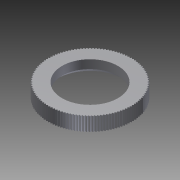
# Autodesk Inventor part: AT504
Saved by Autodesk Inventor 2014 (Build 180170000, 170)
## iProperties
Category: PARTsolutions
Company: NKKSWITCHES
Created: 2013-12-28
Part Number: AT504
Catalog Web Link: www.cadenas.de
Description: AT504 - Knurled Face Nut-
Vendor: NKKSWITCHES
Document SubType Name: Modeling
Designer: PARTuser1
Manufacturer: NKKSWITCHES
Density: 1 g/cm^3
Material: Generic
Appearance: RGB(192.00000375509219,192.00000375509219,192.00000375509219)
PSOL_IDENT_0: {$CADENAS_DATA\23d-libs\nkkswitches\pushbuttons\sb4011\parts\at504.prj},170 {VTYP=3D},{NB=AT504},{LI
PSOL_IDENT_1: NA=AT504},{NN=AT504 - Knurled Face Nut},{DATE=17.02.2009 10:23:06},{GEOMDATE=16.02.2009 13:27:00},{V
PSOL_IDENT_2: ERSION=},{LINEID=10},{LINESUBID=-1},{WBVAR=}  {NB=AT504},{LINA=AT504},{KT=DUMMY},{PN=AT504}
CNS_NN: AT504 - Knurled Face Nut
CNS_NB: AT504
CNS_NBSYN: $PN.
CNS_LINA: AT504
CNS_PN: AT504
SUPPLIER: NKKSWITCHES
ARTICLENO: AT504
BOMINFO: AT504
CREATOR: CADENAS GmbH
Title: AT504
Author: Cadenas PARTsolutions
Autodesk Inventor part; units mm, degrees
sketch "Sketch_1" plane through (0, 0, 0) normal (0, 1, 0) x (-1, 0, 0)
  line L0 (7.5946, 0) -> (7.3635, 0.1928)
  line L1 (7.3635, 0.1928) -> (7.5842, 0.3975)
  line L2 (7.5842, 0.3975) -> (7.3433, 0.5779)
  line L3 (7.3433, 0.5779) -> (7.553, 0.7939)
  line L4 (7.553, 0.7939) -> (7.303, 0.9615)
  line L5 (7.303, 0.9615) -> (7.5011, 1.1881)
  line L6 (7.5011, 1.1881) -> (7.2427, 1.3423)
  line L7 (7.2427, 1.3423) -> (7.4286, 1.579)
  line L8 (7.4286, 1.579) -> (7.1625, 1.7196)
  line L9 (7.1625, 1.7196) -> (7.3358, 1.9656)
  line L10 (7.3358, 1.9656) -> (7.0627, 2.0921)
  line L11 (7.0627, 2.0921) -> (7.2229, 2.3469)
  line L12 (7.2229, 2.3469) -> (6.9435, 2.4588)
  line L13 (6.9435, 2.4588) -> (7.0902, 2.7217)
  line L14 (7.0902, 2.7217) -> (6.8053, 2.8188)
  line L15 (6.8053, 2.8188) -> (6.938, 3.089)
  line L16 (6.938, 3.089) -> (6.6484, 3.1711)
  line L17 (6.6484, 3.1711) -> (6.7668, 3.4479)
  line L18 (6.7668, 3.4479) -> (6.4734, 3.5148)
  line L19 (6.4734, 3.5148) -> (6.5771, 3.7973)
  line L20 (6.5771, 3.7973) -> (6.2805, 3.8487)
  line L21 (6.2805, 3.8487) -> (6.3694, 4.1363)
  line L22 (6.3694, 4.1363) -> (6.0705, 4.1721)
  line L23 (6.0705, 4.1721) -> (6.1442, 4.464)
  line L24 (6.1442, 4.464) -> (5.8438, 4.4841)
  line L25 (5.8438, 4.4841) -> (5.9021, 4.7794)
  line L26 (5.9021, 4.7794) -> (5.6012, 4.7838)
  line L27 (5.6012, 4.7838) -> (5.6439, 5.0818)
  line L28 (5.6439, 5.0818) -> (5.3431, 5.0704)
  line L29 (5.3431, 5.0704) -> (5.3702, 5.3702)
  line L30 (5.3702, 5.3702) -> (5.0704, 5.3431)
  line L31 (5.0704, 5.3431) -> (5.0818, 5.6439)
  line L32 (5.0818, 5.6439) -> (4.7838, 5.6012)
  line L33 (4.7838, 5.6012) -> (4.7794, 5.9021)
  line L34 (4.7794, 5.9021) -> (4.4841, 5.8438)
  line L35 (4.4841, 5.8438) -> (4.464, 6.1442)
  line L36 (4.464, 6.1442) -> (4.1721, 6.0705)
  line L37 (4.1721, 6.0705) -> (4.1363, 6.3694)
  line L38 (4.1363, 6.3694) -> (3.8487, 6.2805)
  line L39 (3.8487, 6.2805) -> (3.7973, 6.5771)
  line L40 (3.7973, 6.5771) -> (3.5148, 6.4734)
  line L41 (3.5148, 6.4734) -> (3.4479, 6.7668)
  line L42 (3.4479, 6.7668) -> (3.1711, 6.6484)
  line L43 (3.1711, 6.6484) -> (3.089, 6.938)
  line L44 (3.089, 6.938) -> (2.8188, 6.8053)
  line L45 (2.8188, 6.8053) -> (2.7217, 7.0902)
  line L46 (2.7217, 7.0902) -> (2.4588, 6.9435)
  line L47 (2.4588, 6.9435) -> (2.3469, 7.2229)
  line L48 (2.3469, 7.2229) -> (2.0921, 7.0627)
  line L49 (2.0921, 7.0627) -> (1.9656, 7.3358)
  line L50 (1.9656, 7.3358) -> (1.7196, 7.1625)
  line L51 (1.7196, 7.1625) -> (1.579, 7.4286)
  line L52 (1.579, 7.4286) -> (1.3423, 7.2427)
  line L53 (1.3423, 7.2427) -> (1.1881, 7.5011)
  line L54 (1.1881, 7.5011) -> (0.9615, 7.303)
  line L55 (0.9615, 7.303) -> (0.7939, 7.553)
  line L56 (0.7939, 7.553) -> (0.5779, 7.3433)
  line L57 (0.5779, 7.3433) -> (0.3975, 7.5842)
  line L58 (0.3975, 7.5842) -> (0.1928, 7.3635)
  line L59 (0.1928, 7.3635) -> (0, 7.5946)
  line L60 (0, 7.5946) -> (-0.1928, 7.3635)
  line L61 (-0.1928, 7.3635) -> (-0.3975, 7.5842)
  line L62 (-0.3975, 7.5842) -> (-0.5779, 7.3433)
  line L63 (-0.5779, 7.3433) -> (-0.7939, 7.553)
  line L64 (-0.7939, 7.553) -> (-0.9615, 7.303)
  line L65 (-0.9615, 7.303) -> (-1.1881, 7.5011)
  line L66 (-1.1881, 7.5011) -> (-1.3423, 7.2427)
  line L67 (-1.3423, 7.2427) -> (-1.579, 7.4286)
  line L68 (-1.579, 7.4286) -> (-1.7196, 7.1625)
  line L69 (-1.7196, 7.1625) -> (-1.9656, 7.3358)
  line L70 (-1.9656, 7.3358) -> (-2.0921, 7.0627)
  line L71 (-2.0921, 7.0627) -> (-2.3469, 7.2229)
  line L72 (-2.3469, 7.2229) -> (-2.4588, 6.9435)
  line L73 (-2.4588, 6.9435) -> (-2.7217, 7.0902)
  line L74 (-2.7217, 7.0902) -> (-2.8188, 6.8053)
  line L75 (-2.8188, 6.8053) -> (-3.089, 6.938)
  line L76 (-3.089, 6.938) -> (-3.1711, 6.6484)
  line L77 (-3.1711, 6.6484) -> (-3.4479, 6.7668)
  line L78 (-3.4479, 6.7668) -> (-3.5148, 6.4734)
  line L79 (-3.5148, 6.4734) -> (-3.7973, 6.5771)
  line L80 (-3.7973, 6.5771) -> (-3.8487, 6.2805)
  line L81 (-3.8487, 6.2805) -> (-4.1363, 6.3694)
  line L82 (-4.1363, 6.3694) -> (-4.1721, 6.0705)
  line L83 (-4.1721, 6.0705) -> (-4.464, 6.1442)
  line L84 (-4.464, 6.1442) -> (-4.4841, 5.8438)
  line L85 (-4.4841, 5.8438) -> (-4.7794, 5.9021)
  line L86 (-4.7794, 5.9021) -> (-4.7838, 5.6012)
  line L87 (-4.7838, 5.6012) -> (-5.0818, 5.6439)
  line L88 (-5.0818, 5.6439) -> (-5.0704, 5.3431)
  line L89 (-5.0704, 5.3431) -> (-5.3702, 5.3702)
  line L90 (-5.3702, 5.3702) -> (-5.3431, 5.0704)
  line L91 (-5.3431, 5.0704) -> (-5.6439, 5.0818)
  line L92 (-5.6439, 5.0818) -> (-5.6012, 4.7838)
  line L93 (-5.6012, 4.7838) -> (-5.9021, 4.7794)
  line L94 (-5.9021, 4.7794) -> (-5.8438, 4.4841)
  line L95 (-5.8438, 4.4841) -> (-6.1442, 4.464)
  line L96 (-6.1442, 4.464) -> (-6.0705, 4.1721)
  line L97 (-6.0705, 4.1721) -> (-6.3694, 4.1363)
  line L98 (-6.3694, 4.1363) -> (-6.2805, 3.8487)
  line L99 (-6.2805, 3.8487) -> (-6.5771, 3.7973)
  line L100 (-6.5771, 3.7973) -> (-6.4734, 3.5148)
  line L101 (-6.4734, 3.5148) -> (-6.7668, 3.4479)
  line L102 (-6.7668, 3.4479) -> (-6.6484, 3.1711)
  line L103 (-6.6484, 3.1711) -> (-6.938, 3.089)
  line L104 (-6.938, 3.089) -> (-6.8053, 2.8188)
  line L105 (-6.8053, 2.8188) -> (-7.0902, 2.7217)
  line L106 (-7.0902, 2.7217) -> (-6.9435, 2.4588)
  line L107 (-6.9435, 2.4588) -> (-7.2229, 2.3469)
  line L108 (-7.2229, 2.3469) -> (-7.0627, 2.0921)
  line L109 (-7.0627, 2.0921) -> (-7.3358, 1.9656)
  line L110 (-7.3358, 1.9656) -> (-7.1625, 1.7196)
  line L111 (-7.1625, 1.7196) -> (-7.4286, 1.579)
  line L112 (-7.4286, 1.579) -> (-7.2427, 1.3423)
  line L113 (-7.2427, 1.3423) -> (-7.5011, 1.1881)
  line L114 (-7.5011, 1.1881) -> (-7.303, 0.9615)
  line L115 (-7.303, 0.9615) -> (-7.553, 0.7939)
  line L116 (-7.553, 0.7939) -> (-7.3433, 0.5779)
  line L117 (-7.3433, 0.5779) -> (-7.5842, 0.3975)
  line L118 (-7.5842, 0.3975) -> (-7.3635, 0.1928)
  line L119 (-7.3635, 0.1928) -> (-7.5946, 0)
  line L120 (-7.5946, 0) -> (-7.3635, -0.1928)
  line L121 (-7.3635, -0.1928) -> (-7.5842, -0.3975)
  line L122 (-7.5842, -0.3975) -> (-7.3433, -0.5779)
  line L123 (-7.3433, -0.5779) -> (-7.553, -0.7939)
  line L124 (-7.553, -0.7939) -> (-7.303, -0.9615)
  line L125 (-7.303, -0.9615) -> (-7.5011, -1.1881)
  line L126 (-7.5011, -1.1881) -> (-7.2427, -1.3423)
  line L127 (-7.2427, -1.3423) -> (-7.4286, -1.579)
  line L128 (-7.4286, -1.579) -> (-7.1625, -1.7196)
  line L129 (-7.1625, -1.7196) -> (-7.3358, -1.9656)
  line L130 (-7.3358, -1.9656) -> (-7.0627, -2.0921)
  line L131 (-7.0627, -2.0921) -> (-7.2229, -2.3469)
  line L132 (-7.2229, -2.3469) -> (-6.9435, -2.4588)
  line L133 (-6.9435, -2.4588) -> (-7.0902, -2.7217)
  line L134 (-7.0902, -2.7217) -> (-6.8053, -2.8188)
  line L135 (-6.8053, -2.8188) -> (-6.938, -3.089)
  line L136 (-6.938, -3.089) -> (-6.6484, -3.1711)
  line L137 (-6.6484, -3.1711) -> (-6.7668, -3.4479)
  line L138 (-6.7668, -3.4479) -> (-6.4734, -3.5148)
  line L139 (-6.4734, -3.5148) -> (-6.5771, -3.7973)
  line L140 (-6.5771, -3.7973) -> (-6.2805, -3.8487)
  line L141 (-6.2805, -3.8487) -> (-6.3694, -4.1363)
  line L142 (-6.3694, -4.1363) -> (-6.0705, -4.1721)
  line L143 (-6.0705, -4.1721) -> (-6.1442, -4.464)
  line L144 (-6.1442, -4.464) -> (-5.8438, -4.4841)
  line L145 (-5.8438, -4.4841) -> (-5.9021, -4.7794)
  line L146 (-5.9021, -4.7794) -> (-5.6012, -4.7838)
  line L147 (-5.6012, -4.7838) -> (-5.6439, -5.0818)
  line L148 (-5.6439, -5.0818) -> (-5.3431, -5.0704)
  line L149 (-5.3431, -5.0704) -> (-5.3702, -5.3702)
  line L150 (-5.3702, -5.3702) -> (-5.0704, -5.3431)
  line L151 (-5.0704, -5.3431) -> (-5.0818, -5.6439)
  line L152 (-5.0818, -5.6439) -> (-4.7838, -5.6012)
  line L153 (-4.7838, -5.6012) -> (-4.7794, -5.9021)
  line L154 (-4.7794, -5.9021) -> (-4.4841, -5.8438)
  line L155 (-4.4841, -5.8438) -> (-4.464, -6.1442)
  line L156 (-4.464, -6.1442) -> (-4.1721, -6.0705)
  line L157 (-4.1721, -6.0705) -> (-4.1363, -6.3694)
  line L158 (-4.1363, -6.3694) -> (-3.8487, -6.2805)
  line L159 (-3.8487, -6.2805) -> (-3.7973, -6.5771)
  line L160 (-3.7973, -6.5771) -> (-3.5148, -6.4734)
  line L161 (-3.5148, -6.4734) -> (-3.4479, -6.7668)
  line L162 (-3.4479, -6.7668) -> (-3.1711, -6.6484)
  line L163 (-3.1711, -6.6484) -> (-3.089, -6.938)
  line L164 (-3.089, -6.938) -> (-2.8188, -6.8053)
  line L165 (-2.8188, -6.8053) -> (-2.7217, -7.0902)
  line L166 (-2.7217, -7.0902) -> (-2.4588, -6.9435)
  line L167 (-2.4588, -6.9435) -> (-2.3469, -7.2229)
  line L168 (-2.3469, -7.2229) -> (-2.0921, -7.0627)
  line L169 (-2.0921, -7.0627) -> (-1.9656, -7.3358)
  line L170 (-1.9656, -7.3358) -> (-1.7196, -7.1625)
  line L171 (-1.7196, -7.1625) -> (-1.579, -7.4286)
  line L172 (-1.579, -7.4286) -> (-1.3423, -7.2427)
  line L173 (-1.3423, -7.2427) -> (-1.1881, -7.5011)
  line L174 (-1.1881, -7.5011) -> (-0.9615, -7.303)
  line L175 (-0.9615, -7.303) -> (-0.7939, -7.553)
  line L176 (-0.7939, -7.553) -> (-0.5779, -7.3433)
  line L177 (-0.5779, -7.3433) -> (-0.3975, -7.5842)
  line L178 (-0.3975, -7.5842) -> (-0.1928, -7.3635)
  line L179 (-0.1928, -7.3635) -> (0, -7.5946)
  line L180 (0, -7.5946) -> (0.1928, -7.3635)
  line L181 (0.1928, -7.3635) -> (0.3975, -7.5842)
  line L182 (0.3975, -7.5842) -> (0.5779, -7.3433)
  line L183 (0.5779, -7.3433) -> (0.7939, -7.553)
  line L184 (0.7939, -7.553) -> (0.9615, -7.303)
  line L185 (0.9615, -7.303) -> (1.1881, -7.5011)
  line L186 (1.1881, -7.5011) -> (1.3423, -7.2427)
  line L187 (1.3423, -7.2427) -> (1.579, -7.4286)
  line L188 (1.579, -7.4286) -> (1.7196, -7.1625)
  line L189 (1.7196, -7.1625) -> (1.9656, -7.3358)
  line L190 (1.9656, -7.3358) -> (2.0921, -7.0627)
  line L191 (2.0921, -7.0627) -> (2.3469, -7.2229)
  line L192 (2.3469, -7.2229) -> (2.4588, -6.9435)
  line L193 (2.4588, -6.9435) -> (2.7217, -7.0902)
  line L194 (2.7217, -7.0902) -> (2.8188, -6.8053)
  line L195 (2.8188, -6.8053) -> (3.089, -6.938)
  line L196 (3.089, -6.938) -> (3.1711, -6.6484)
  line L197 (3.1711, -6.6484) -> (3.4479, -6.7668)
  line L198 (3.4479, -6.7668) -> (3.5148, -6.4734)
  line L199 (3.5148, -6.4734) -> (3.7973, -6.5771)
  line L200 (3.7973, -6.5771) -> (3.8487, -6.2805)
  line L201 (3.8487, -6.2805) -> (4.1363, -6.3694)
  line L202 (4.1363, -6.3694) -> (4.1721, -6.0705)
  line L203 (4.1721, -6.0705) -> (4.464, -6.1442)
  line L204 (4.464, -6.1442) -> (4.4841, -5.8438)
  line L205 (4.4841, -5.8438) -> (4.7794, -5.9021)
  line L206 (4.7794, -5.9021) -> (4.7838, -5.6012)
  line L207 (4.7838, -5.6012) -> (5.0818, -5.6439)
  line L208 (5.0818, -5.6439) -> (5.0704, -5.3431)
  line L209 (5.0704, -5.3431) -> (5.3702, -5.3702)
  line L210 (5.3702, -5.3702) -> (5.3431, -5.0704)
  line L211 (5.3431, -5.0704) -> (5.6439, -5.0818)
  line L212 (5.6439, -5.0818) -> (5.6012, -4.7838)
  line L213 (5.6012, -4.7838) -> (5.9021, -4.7794)
  line L214 (5.9021, -4.7794) -> (5.8438, -4.4841)
  line L215 (5.8438, -4.4841) -> (6.1442, -4.464)
  line L216 (6.1442, -4.464) -> (6.0705, -4.1721)
  line L217 (6.0705, -4.1721) -> (6.3694, -4.1363)
  line L218 (6.3694, -4.1363) -> (6.2805, -3.8487)
  line L219 (6.2805, -3.8487) -> (6.5771, -3.7973)
  line L220 (6.5771, -3.7973) -> (6.4734, -3.5148)
  line L221 (6.4734, -3.5148) -> (6.7668, -3.4479)
  line L222 (6.7668, -3.4479) -> (6.6484, -3.1711)
  line L223 (6.6484, -3.1711) -> (6.938, -3.089)
  line L224 (6.938, -3.089) -> (6.8053, -2.8188)
  line L225 (6.8053, -2.8188) -> (7.0902, -2.7217)
  line L226 (7.0902, -2.7217) -> (6.9435, -2.4588)
  line L227 (6.9435, -2.4588) -> (7.2229, -2.3469)
  line L228 (7.2229, -2.3469) -> (7.0627, -2.0921)
  line L229 (7.0627, -2.0921) -> (7.3358, -1.9656)
  line L230 (7.3358, -1.9656) -> (7.1625, -1.7196)
  line L231 (7.1625, -1.7196) -> (7.4286, -1.579)
  line L232 (7.4286, -1.579) -> (7.2427, -1.3423)
  line L233 (7.2427, -1.3423) -> (7.5011, -1.1881)
  line L234 (7.5011, -1.1881) -> (7.303, -0.9615)
  line L235 (7.303, -0.9615) -> (7.553, -0.7939)
  line L236 (7.553, -0.7939) -> (7.3433, -0.5779)
  line L237 (7.3433, -0.5779) -> (7.5842, -0.3975)
  line L238 (7.5842, -0.3975) -> (7.3635, -0.1928)
  line L239 (7.3635, -0.1928) -> (7.5946, 0)
  constraints: 480 end point
extrude "Extrusion1" add sketch "Sketch_1" along normal blind 2.4892
sketch "Sketch2" plane through (0, 0, 0) normal (0, -1, 0) x (1, 0, 0)
  point P0 (0, 0)
hole "Drilling 1" at (0, 0, 0) direction (0, 1, 0) diameter 10.106 depth 2.4892 countersink diameter 12 countersink angle 90
ref_plane "1_XY" through (0, 0, 0) normal (0, 1, 0) x (1, 0, 0)
ref_plane "1_YZ" through (0, 0, 0) normal (1, 0, 0) x (0, 0, -1)
ref_plane "1_ZX" through (0, 0, 0) normal (0, 0, -1) x (0, 1, 0)
body "Solid1"
